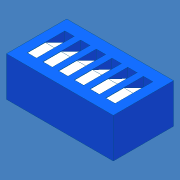
# Autodesk Inventor part: cRIO-FRC DIP Switch
Saved by Autodesk Inventor 2011 (Build 150239000, 239)
## iProperties
Category: FRC Parts
Manager: Ed Sparks
Company: FirstCadLibrary
Shininess: 64.0
Length Units: 11272
Angle Units: 11279
Time Units: 11290
Mass Units: 11286
Length Display Precision: 3
Angle Display Precision: 2
Compacted: True
Part Number: cRIO-FRC DIP Switch
Document SubType Name: Modeling
Created: 2005-12-26
Designer: Ed Sparks
Material: ABS Plastic
Project: FIRST
Engineer: Ed Sparks
Density: 1 g/cm^3
Density: 0.0
Volumn: 0.0
Area: 0.0
PropertySet Name: Model Information
Control State: 0
Master: False
Checked Out: False
Author: Ed Sparks
Keywords: FIRST
Autodesk Inventor part; units mm, degrees
ref_plane "YZ Plane" through (0, 0, 0) normal (1, 0, 0) x (0, 1, 0)
ref_plane "XZ Plane" through (0, 0, 0) normal (0, 1, 0) x (-1, 0, 0)
ref_plane "XY Plane" through (0, 0, 0) normal (0, 0, 1) x (1, 0, 0)
sketch "Sketch1" plane through (0, 0, 0) normal (0, 0, 1) x (1, 0, 0)
  line L0 (0, 0) -> (17.272, 0)
  line L1 (17.272, 0) -> (17.272, 9.7409)
  line L2 (17.272, 9.7409) -> (0, 9.7409)
  line L3 (0, 9.7409) -> (0, 0)
  dimension "d0" = 9.7409
  dimension "d1" = 17.272
  constraints: 8 end point, 2 parallel, 1 horizontal, 1 perpendicular, 1 other
  measures "d0" distance of L2.end L0.start
  measures "d1" distance of L1.end L2.end
extrude "Extrusion1" add sketch "Sketch1" along normal blind 6.3881
sketch "Sketch2" plane through (0, 0, 6.3881) normal (0, 0, 1) x (1, 0, 0)
  line L0 (0, 0) -> (0, 9.7409)
  line L1 (17.272, 0) -> (0, 0)
  line L2 (0, 9.7409) -> (17.272, 9.7409)
  line L3 (1.524, 7.9185) -> (3.048, 7.9185)
  line L4 (3.048, 7.9185) -> (3.048, 1.8225)
  line L5 (3.048, 1.8225) -> (1.524, 1.8224)
  line L6 (1.524, 1.8224) -> (1.524, 7.9185)
  line L7 (3.048, 7.9185) -> (3.048, 9.7409)
  line L8 (1.524, 1.8224) -> (1.524, 0)
  dimension "d4" = 1.524
  dimension "d5" = 6.096
  dimension "d7" = 1.524
  constraints: 12 end point, 3 parallel, 3 perpendicular, 2 point on line, 1 horizontal
  measures "d4" distance of L3.start L3.end
  measures "d5" distance of L3.end L4.end
  measures "d7" distance between parallel lines of L6 L0
extrude "Extrusion2" cut sketch "Sketch2" against normal blind 2.54 contours L6 L3 L4 L5
sketch "Sketch6" plane through (0, 0, 3.8481) normal (0, 0, 1) x (1, 0, 0)
  line L0 (1.524, 1.8224) -> (3.048, 1.8225)
  line L1 (3.048, 1.8225) -> (3.048, 7.9185)
  line L2 (3.048, 7.9185) -> (1.524, 7.9185)
  line L3 (1.524, 7.9185) -> (1.524, 1.8224)
  line L4 (1.5494, 7.9185) -> (3.0226, 7.9184)
  line L5 (3.0226, 7.9184) -> (3.0226, 1.8225)
  line L6 (3.0226, 1.8225) -> (1.5494, 1.8224)
  line L7 (1.5494, 1.8224) -> (1.5494, 7.9185)
  line L8 (1.5494, 4.8704) -> (1.524, 4.8705) construction
  line L9 (3.0226, 4.8704) -> (3.048, 4.8704) construction
  dimension "d38" = 0.0254
  constraints: 12 end point, 4 midpoint, 2 parallel, 2 point on line, 1 collinear, 1 horizontal, 1 perpendicular
  measures "d38" distance between parallel lines of L3 L7
extrude "Extrusion6" add sketch "Sketch6" along normal blind 2.5146 contours L7 L2 L5 L0
sketch "Sketch7" plane through (3.0226, 1.8225, 3.8481) normal (1, 0, 0) x (0, 0, -1)
  line L0 (-2.5146, 6.096) -> (-2.5146, 0) projected
  line L1 (-2.5146, 6.096) -> (0, 6.096) projected
  line L2 (-0.9525, 6.096) -> (-2.5146, 2.921)
  point P0 (-2.54, 6.096)
  dimension "d41" = 3.175
  dimension "d42" = 1.5875
  constraints: 2 end point, 2 point on line
  measures "d41" distance from line of L2.end L1
  measures "d42" distance of L2.start point (-2.54, 6.096)
extrude "Extrusion7" cut sketch "Sketch7" against normal up to surface (1.4986 mm away)
pattern_linear "Rectangular Pattern5" count 6 spacing 2.54 along (1, 0, 0) of "Extrusion2"
pattern_linear "Rectangular Pattern6" count 6 spacing 2.54 along (1, 0, 0) of "Extrusion6", "Extrusion7"
body "Solid1"
